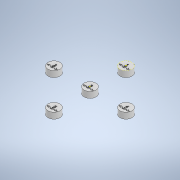
# Autodesk Inventor part: 5-circles-test-print
Saved by Autodesk Inventor 2020.3 (Build 243373000, 373)
## iProperties
Created: 2020-06-02
Part Number: 5-circles-test-print
Material: Generic
Document SubType Name: Modeling
Designer: robst
Density: 1 g/cm^3
Appearance: Default
Author: robst
Autodesk Inventor part; units mm, degrees
ref_plane "YZ Plane" through (0, 0, 0) normal (1, 0, 0) x (0, 1, 0)
ref_plane "XZ Plane" through (0, 0, 0) normal (0, 1, 0) x (-1, 0, 0)
ref_plane "XY Plane" through (0, 0, 0) normal (0, 0, 1) x (1, 0, 0)
sketch "Sketch1" plane through (0, 0, 0) normal (0, 1, 0) x (-1, 0, 0)
  circle A0 centre (0, 0) radius 12.7
  circle A1 centre (76.2, 0) radius 12.7
  circle A2 centre (0, -76.2) radius 12.7
  circle A3 centre (-76.2, 0) radius 12.7
  circle A4 centre (0, 76.2) radius 12.7
  dimension "d0" = 25.4
  dimension "d1" = 76.2
  dimension "d2" = 76.2
  dimension "d3" = 76.2
  dimension "d4" = 76.2
  constraints: 5 centre point, 4 equal radius, 1 coincident
  measures "d0" diameter of A0
  measures "d1" distance of A1.centre point (0, 0)
  measures "d2" distance of A2.centre point (0, 0)
  measures "d3" distance of A3.centre point (0, 0)
  measures "d4" distance of A4.centre point (0, 0)
extrude "Extrusion1" add sketch "Sketch1" along normal blind 12.7
sketch "Sketch4" plane through (0, 12.7, -76.2) normal (0, 1, 0) x (1, 0, 0)
  circle A0 centre (0, 0) radius 12.7 construction
  point P0 (0, -76.2)
sketch "Sketch5" plane through (0, 12.7, 0) normal (0, 1, 0) x (1, 0, 0)
  circle A0 centre (0, 76.2) radius 12.7 construction
  line L0 (-12.7, 76.2) -> (12.7, 76.2) construction
  circle A1 centre (0, 0) radius 12.7 construction
  line L1 (-12.7, 0) -> (12.7, 0) construction
  line L2 (-88.5573, 0) -> (-63.5, 0) construction
  circle A2 centre (-76.2, 0) radius 12.7 construction
  circle A3 centre (76.2, 0) radius 12.7 construction
  line L3 (63.5, 0) -> (88.9, 0) construction
  circle A4 centre (0, -76.2) radius 12.7 construction
  line L4 (-12.7, -76.2) -> (12.7, -76.2) construction
  line L5 (1.7969, 76.2) -> (-1.5582, 76.2)
  line L6 (-1.5582, 76.2) -> (-1.5582, 77.0851)
  line L7 (-1.5582, 77.0851) -> (-0.4878, 77.0851)
  line L8 (-0.4878, 77.0851) -> (-0.4878, 79.7733)
  line L9 (-0.4878, 79.7733) -> (-1.5582, 79.7733)
  line L10 (-1.5582, 79.7733) -> (-1.5582, 80.6007)
  spline S0 degree 2 poles (-1.5582, 80.6007) (-1.3235, 80.6007) (-0.8583, 80.6625) (-0.7184, 80.7284) knots 0 0 0 1 2 2 2
  spline S1 degree 2 poles (-0.7184, 80.7284) (-0.5578, 80.8107) (-0.3767, 81.0865) (-0.3602, 81.2924) knots 0 0 0 1 2 2 2
  line L11 (-0.3602, 81.2924) -> (0.7513, 81.2924)
  line L12 (0.7513, 81.2924) -> (0.7513, 77.0851)
  line L13 (0.7513, 77.0851) -> (1.7969, 77.0851)
  line L14 (1.7969, 77.0851) -> (1.7969, 76.2)
  line L15 (-6.1256, 70.1534) -> (-10.5058, 71.973)
  line L16 (-10.5058, 71.973) -> (-10.5058, 72.7222)
  line L17 (-10.5058, 72.7222) -> (-6.1256, 74.5418)
  line L18 (-6.1256, 74.5418) -> (-6.1256, 73.5991)
  line L19 (-6.1256, 73.5991) -> (-9.1885, 72.3435)
  line L20 (-9.1885, 72.3435) -> (-6.1256, 71.0961)
  line L21 (-6.1256, 71.0961) -> (-6.1256, 70.1534)
  line L22 (-2.7705, 71.8742) -> (-5.0306, 71.8742)
  line L23 (-5.0306, 71.8742) -> (-5.0306, 72.821)
  line L24 (-5.0306, 72.821) -> (-2.7705, 72.821)
  line L25 (-2.7705, 72.821) -> (-2.7705, 71.8742)
  line L26 (2.433, 70.104) -> (0.9592, 70.104)
  line L27 (0.9592, 70.104) -> (-0.0206, 71.7219)
  line L28 (-0.0206, 71.7219) -> (-1.0209, 70.104)
  line L29 (-1.0209, 70.104) -> (-2.433, 70.104)
  line L30 (-2.433, 70.104) -> (-0.7822, 72.6605)
  line L31 (-0.7822, 72.6605) -> (-2.3671, 75.184)
  line L32 (-2.3671, 75.184) -> (-0.8933, 75.184)
  line L33 (-0.8933, 75.184) -> (0.0247, 73.6485)
  line L34 (0.0247, 73.6485) -> (0.9674, 75.184)
  line L35 (0.9674, 75.184) -> (2.3794, 75.184)
  line L36 (2.3794, 75.184) -> (0.7863, 72.714)
  line L37 (0.7863, 72.714) -> (2.433, 70.104)
  line L38 (5.1088, 71.8742) -> (2.8488, 71.8742)
  line L39 (2.8488, 71.8742) -> (2.8488, 72.821)
  line L40 (2.8488, 72.821) -> (5.1088, 72.821)
  line L41 (5.1088, 72.821) -> (5.1088, 71.8742)
  line L42 (10.5881, 71.973) -> (6.208, 70.1534)
  line L43 (6.208, 70.1534) -> (6.208, 71.0961)
  line L44 (6.208, 71.0961) -> (9.2667, 72.3476)
  line L45 (9.2667, 72.3476) -> (6.208, 73.5991)
  line L46 (6.208, 73.5991) -> (6.208, 74.5418)
  line L47 (6.208, 74.5418) -> (10.5881, 72.7222)
  line L48 (10.5881, 72.7222) -> (10.5881, 71.973)
  line L49 (-74.0053, 0) -> (-77.7391, 0)
  line L50 (-77.7391, 0) -> (-77.7391, 0.8275)
  spline S2 degree 2 poles (-77.7391, 0.8275) (-77.2657, 1.2062) (-76.5082, 1.8731) (-76.2242, 2.1736) knots 0 0 0 1 2 2 2
  spline S3 degree 2 poles (-76.2242, 2.1736) (-75.8496, 2.5647) (-75.5161, 3.1616) (-75.5161, 3.4745) knots 0 0 0 1 2 2 2
  spline S4 degree 2 poles (-75.5161, 3.4745) (-75.5161, 3.8285) (-75.9401, 4.2073) (-76.3189, 4.2073) knots 0 0 0 1 2 2 2
  spline S5 degree 2 poles (-76.3189, 4.2073) (-76.5124, 4.2073) (-76.8582, 4.1126) (-77.0352, 4.0385) knots 0 0 0 1 2 2 2
  spline S6 degree 2 poles (-77.0352, 4.0385) (-77.2081, 3.9603) (-77.4551, 3.7956) (-77.5168, 3.7544) knots 0 0 0 1 2 2 2
  line L51 (-77.5168, 3.7544) -> (-77.6156, 3.7544)
  line L52 (-77.6156, 3.7544) -> (-77.6156, 4.8618)
  spline S7 degree 2 poles (-77.6156, 4.8618) (-77.4016, 4.9647) (-76.4877, 5.1788) (-76.0636, 5.1788) knots 0 0 0 1 2 2 2
  spline S8 degree 2 poles (-76.0636, 5.1788) (-75.158, 5.1788) (-74.2276, 4.3719) (-74.2276, 3.6433) knots 0 0 0 1 2 2 2
  spline S9 degree 2 poles (-74.2276, 3.6433) (-74.2276, 3.1946) (-74.6516, 2.33) (-75.1415, 1.836) knots 0 0 0 1 2 2 2
  spline S10 degree 2 poles (-75.1415, 1.836) (-75.4502, 1.5314) (-76.0307, 1.058) (-76.1583, 0.9592) knots 0 0 0 1 2 2 2
  line L53 (-76.1583, 0.9592) -> (-74.0053, 0.9592)
  line L54 (-74.0053, 0.9592) -> (-74.0053, 0)
  line L55 (-82.1543, -6.0466) -> (-86.5344, -4.227)
  line L56 (-86.5344, -4.227) -> (-86.5344, -3.4778)
  line L57 (-86.5344, -3.4778) -> (-82.1543, -1.6582)
  line L58 (-82.1543, -1.6582) -> (-82.1543, -2.6009)
  line L59 (-82.1543, -2.6009) -> (-85.2171, -3.8565)
  line L60 (-85.2171, -3.8565) -> (-82.1543, -5.1039)
  line L61 (-82.1543, -5.1039) -> (-82.1543, -6.0466)
  line L62 (-78.7992, -4.3258) -> (-81.0592, -4.3258)
  line L63 (-81.0592, -4.3258) -> (-81.0592, -3.379)
  line L64 (-81.0592, -3.379) -> (-78.7992, -3.379)
  line L65 (-78.7992, -3.379) -> (-78.7992, -4.3258)
  line L66 (-73.5957, -6.096) -> (-75.0695, -6.096)
  line L67 (-75.0695, -6.096) -> (-76.0492, -4.4781)
  line L68 (-76.0492, -4.4781) -> (-77.0496, -6.096)
  line L69 (-77.0496, -6.096) -> (-78.4616, -6.096)
  line L70 (-78.4616, -6.096) -> (-76.8108, -3.5395)
  line L71 (-76.8108, -3.5395) -> (-78.3957, -1.016)
  line L72 (-78.3957, -1.016) -> (-76.922, -1.016)
  line L73 (-76.922, -1.016) -> (-76.0039, -2.5515)
  line L74 (-76.0039, -2.5515) -> (-75.0612, -1.016)
  line L75 (-75.0612, -1.016) -> (-73.6492, -1.016)
  line L76 (-73.6492, -1.016) -> (-75.2424, -3.486)
  line L77 (-75.2424, -3.486) -> (-73.5957, -6.096)
  line L78 (-70.9198, -4.3258) -> (-73.1799, -4.3258)
  line L79 (-73.1799, -4.3258) -> (-73.1799, -3.379)
  line L80 (-73.1799, -3.379) -> (-70.9198, -3.379)
  line L81 (-70.9198, -3.379) -> (-70.9198, -4.3258)
  line L82 (-65.4405, -4.227) -> (-69.8207, -6.0466)
  line L83 (-69.8207, -6.0466) -> (-69.8207, -5.1039)
  line L84 (-69.8207, -5.1039) -> (-66.762, -3.8524)
  line L85 (-66.762, -3.8524) -> (-69.8207, -2.6009)
  line L86 (-69.8207, -2.6009) -> (-69.8207, -1.6582)
  line L87 (-69.8207, -1.6582) -> (-65.4405, -3.4778)
  line L88 (-65.4405, -3.4778) -> (-65.4405, -4.227)
  spline S11 degree 2 poles (1.8957, 1.5396) (1.8957, 1.165) (1.6199, 0.5516) (1.3523, 0.3376) knots 0 0 0 1 2 2 2
  spline S12 degree 2 poles (1.3523, 0.3376) (1.0847, 0.1235) (0.3561, -0.107) (-0.1667, -0.107) knots 0 0 0 1 2 2 2
  spline S13 degree 2 poles (-0.1667, -0.107) (-0.7595, -0.107) (-1.6076, 0.0906) (-1.8752, 0.2141) knots 0 0 0 1 2 2 2
  line L89 (-1.8752, 0.2141) -> (-1.8752, 1.3173)
  line L90 (-1.8752, 1.3173) -> (-1.7517, 1.3173)
  spline S14 degree 2 poles (-1.7517, 1.3173) (-1.4717, 1.1403) (-0.7184, 0.8769) (-0.4055, 0.8769) knots 0 0 0 1 2 2 2
  spline S15 degree 2 poles (-0.4055, 0.8769) (-0.2202, 0.8769) (0.212, 0.9427) (0.3602, 1.0498) knots 0 0 0 1 2 2 2
  spline S16 degree 2 poles (0.3602, 1.0498) (0.4755, 1.1362) (0.6154, 1.3873) (0.6154, 1.6137) knots 0 0 0 1 2 2 2
  spline S17 degree 2 poles (0.6154, 1.6137) (0.6154, 1.8402) (0.4178, 2.083) (0.2532, 2.1407) knots 0 0 0 1 2 2 2
  spline S18 degree 2 poles (0.2532, 2.1407) (0.0885, 2.1983) (-0.3684, 2.2107) (-0.5455, 2.2107) knots 0 0 0 1 2 2 2
  line L91 (-0.5455, 2.2107) -> (-0.7636, 2.2107)
  line L92 (-0.7636, 2.2107) -> (-0.7636, 3.104)
  line L93 (-0.7636, 3.104) -> (-0.5619, 3.104)
  spline S19 degree 2 poles (-0.5619, 3.104) (-0.3314, 3.104) (0.0597, 3.1452) (0.1955, 3.2069) knots 0 0 0 1 2 2 2
  spline S20 degree 2 poles (0.1955, 3.2069) (0.3314, 3.2728) (0.4837, 3.5033) (0.4837, 3.7009) knots 0 0 0 1 2 2 2
  spline S21 degree 2 poles (0.4837, 3.7009) (0.4837, 3.8573) (0.3396, 4.0508) (0.2367, 4.1043) knots 0 0 0 1 2 2 2
  spline S22 degree 2 poles (0.2367, 4.1043) (0.1132, 4.1661) (-0.2161, 4.2073) (-0.3314, 4.2073) knots 0 0 0 1 2 2 2
  spline S23 degree 2 poles (-0.3314, 4.2073) (-0.5166, 4.2073) (-0.9077, 4.1208) (-1.0889, 4.0508) knots 0 0 0 1 2 2 2
  spline S24 degree 2 poles (-1.0889, 4.0508) (-1.2329, 3.9973) (-1.5458, 3.8244) (-1.6199, 3.7791) knots 0 0 0 1 2 2 2
  line L94 (-1.6199, 3.7791) -> (-1.727, 3.7791)
  line L95 (-1.727, 3.7791) -> (-1.727, 4.8659)
  spline S25 degree 2 poles (-1.727, 4.8659) (-1.4635, 4.9771) (-0.5743, 5.187) (-0.1091, 5.187) knots 0 0 0 1 2 2 2
  spline S26 degree 2 poles (-0.1091, 5.187) (0.3437, 5.187) (1.0106, 5.0306) (1.2453, 4.8783) knots 0 0 0 1 2 2 2
  spline S27 degree 2 poles (1.2453, 4.8783) (1.5047, 4.7177) (1.764, 4.2237) (1.764, 3.915) knots 0 0 0 1 2 2 2
  spline S28 degree 2 poles (1.764, 3.915) (1.764, 3.4786) (1.2618, 2.8282) (0.8501, 2.7335) knots 0 0 0 1 2 2 2
  line L96 (0.8501, 2.7335) -> (0.8501, 2.6841)
  spline S29 degree 2 poles (0.8501, 2.6841) (1.0312, 2.6594) (1.377, 2.5276) (1.5417, 2.3794) knots 0 0 0 1 2 2 2
  spline S30 degree 2 poles (1.5417, 2.3794) (1.694, 2.2477) (1.8957, 1.8278) (1.8957, 1.5396) knots 0 0 0 1 2 2 2
  line L97 (-6.1256, -6.0466) -> (-10.5058, -4.227)
  line L98 (-10.5058, -4.227) -> (-10.5058, -3.4778)
  line L99 (-10.5058, -3.4778) -> (-6.1256, -1.6582)
  line L100 (-6.1256, -1.6582) -> (-6.1256, -2.6009)
  line L101 (-6.1256, -2.6009) -> (-9.1885, -3.8565)
  line L102 (-9.1885, -3.8565) -> (-6.1256, -5.1039)
  line L103 (-6.1256, -5.1039) -> (-6.1256, -6.0466)
  line L104 (-2.7705, -4.3258) -> (-5.0306, -4.3258)
  line L105 (-5.0306, -4.3258) -> (-5.0306, -3.379)
  line L106 (-5.0306, -3.379) -> (-2.7705, -3.379)
  line L107 (-2.7705, -3.379) -> (-2.7705, -4.3258)
  line L108 (2.433, -6.096) -> (0.9592, -6.096)
  line L109 (0.9592, -6.096) -> (-0.0206, -4.4781)
  line L110 (-0.0206, -4.4781) -> (-1.0209, -6.096)
  line L111 (-1.0209, -6.096) -> (-2.433, -6.096)
  line L112 (-2.433, -6.096) -> (-0.7822, -3.5395)
  line L113 (-0.7822, -3.5395) -> (-2.3671, -1.016)
  line L114 (-2.3671, -1.016) -> (-0.8933, -1.016)
  line L115 (-0.8933, -1.016) -> (0.0247, -2.5515)
  line L116 (0.0247, -2.5515) -> (0.9674, -1.016)
  line L117 (0.9674, -1.016) -> (2.3794, -1.016)
  line L118 (2.3794, -1.016) -> (0.7863, -3.486)
  line L119 (0.7863, -3.486) -> (2.433, -6.096)
  line L120 (5.1088, -4.3258) -> (2.8488, -4.3258)
  line L121 (2.8488, -4.3258) -> (2.8488, -3.379)
  line L122 (2.8488, -3.379) -> (5.1088, -3.379)
  line L123 (5.1088, -3.379) -> (5.1088, -4.3258)
  line L124 (10.5881, -4.227) -> (6.208, -6.0466)
  line L125 (6.208, -6.0466) -> (6.208, -5.1039)
  line L126 (6.208, -5.1039) -> (9.2667, -3.8524)
  line L127 (9.2667, -3.8524) -> (6.208, -2.6009)
  line L128 (6.208, -2.6009) -> (6.208, -1.6582)
  line L129 (6.208, -1.6582) -> (10.5881, -3.4778)
  line L130 (10.5881, -3.4778) -> (10.5881, -4.227)
  line L131 (78.2851, 1.1856) -> (77.5976, 1.1856)
  line L132 (77.5976, 1.1856) -> (77.5976, -0.0124)
  line L133 (77.5976, -0.0124) -> (76.3667, -0.0124)
  line L134 (76.3667, -0.0124) -> (76.3667, 1.1856)
  line L135 (76.3667, 1.1856) -> (74.1272, 1.1856)
  line L136 (74.1272, 1.1856) -> (74.1272, 2.1324)
  line L137 (74.1272, 2.1324) -> (76.3256, 5.08)
  line L138 (76.3256, 5.08) -> (77.5976, 5.08)
  line L139 (77.5976, 5.08) -> (77.5976, 2.0995)
  line L140 (77.5976, 2.0995) -> (78.2851, 2.0995)
  line L141 (78.2851, 2.0995) -> (78.2851, 1.1856)
  line L142 (76.3667, 2.0995) -> (76.3667, 3.8285)
  line L143 (76.3667, 3.8285) -> (75.0782, 2.0995)
  line L144 (75.0782, 2.0995) -> (76.3667, 2.0995)
  line L145 (70.0744, -6.0466) -> (65.6942, -4.227)
  line L146 (65.6942, -4.227) -> (65.6942, -3.4778)
  line L147 (65.6942, -3.4778) -> (70.0744, -1.6582)
  line L148 (70.0744, -1.6582) -> (70.0744, -2.6009)
  line L149 (70.0744, -2.6009) -> (67.0115, -3.8565)
  line L150 (67.0115, -3.8565) -> (70.0744, -5.1039)
  line L151 (70.0744, -5.1039) -> (70.0744, -6.0466)
  line L152 (73.4295, -4.3258) -> (71.1694, -4.3258)
  line L153 (71.1694, -4.3258) -> (71.1694, -3.379)
  line L154 (71.1694, -3.379) -> (73.4295, -3.379)
  line L155 (73.4295, -3.379) -> (73.4295, -4.3258)
  line L156 (78.633, -6.096) -> (77.1592, -6.096)
  line L157 (77.1592, -6.096) -> (76.1794, -4.4781)
  line L158 (76.1794, -4.4781) -> (75.1791, -6.096)
  line L159 (75.1791, -6.096) -> (73.767, -6.096)
  line L160 (73.767, -6.096) -> (75.4178, -3.5395)
  line L161 (75.4178, -3.5395) -> (73.8329, -1.016)
  line L162 (73.8329, -1.016) -> (75.3067, -1.016)
  line L163 (75.3067, -1.016) -> (76.2247, -2.5515)
  line L164 (76.2247, -2.5515) -> (77.1674, -1.016)
  line L165 (77.1674, -1.016) -> (78.5794, -1.016)
  line L166 (78.5794, -1.016) -> (76.9863, -3.486)
  line L167 (76.9863, -3.486) -> (78.633, -6.096)
  line L168 (81.3088, -4.3258) -> (79.0488, -4.3258)
  line L169 (79.0488, -4.3258) -> (79.0488, -3.379)
  line L170 (79.0488, -3.379) -> (81.3088, -3.379)
  line L171 (81.3088, -3.379) -> (81.3088, -4.3258)
  line L172 (86.7881, -4.227) -> (82.408, -6.0466)
  line L173 (82.408, -6.0466) -> (82.408, -5.1039)
  line L174 (82.408, -5.1039) -> (85.4667, -3.8524)
  line L175 (85.4667, -3.8524) -> (82.408, -2.6009)
  line L176 (82.408, -2.6009) -> (82.408, -1.6582)
  line L177 (82.408, -1.6582) -> (86.7881, -3.4778)
  line L178 (86.7881, -3.4778) -> (86.7881, -4.227)
  spline S31 degree 2 poles (1.9081, -74.4792) (1.9081, -74.8785) (1.6364, -75.5537) (1.3688, -75.7966) knots 0 0 0 1 2 2 2
  spline S32 degree 2 poles (1.3688, -75.7966) (1.1012, -76.0394) (0.3684, -76.307) (-0.1667, -76.307) knots 0 0 0 1 2 2 2
  spline S33 degree 2 poles (-0.1667, -76.307) (-0.7348, -76.3029) (-1.5499, -76.1177) (-1.8175, -75.9983) knots 0 0 0 1 2 2 2
  line L179 (-1.8175, -75.9983) -> (-1.8175, -74.8909)
  line L180 (-1.8175, -74.8909) -> (-1.7023, -74.8909)
  spline S34 degree 2 poles (-1.7023, -74.8909) (-1.6035, -74.9444) (-1.3647, -75.0844) (-1.1712, -75.1585) knots 0 0 0 1 2 2 2
  spline S35 degree 2 poles (-1.1712, -75.1585) (-0.9901, -75.2285) (-0.6154, -75.3231) (-0.389, -75.3231) knots 0 0 0 1 2 2 2
  spline S36 degree 2 poles (-0.389, -75.3231) (-0.1914, -75.3231) (0.2696, -75.2243) (0.4096, -75.0926) knots 0 0 0 1 2 2 2
  spline S37 degree 2 poles (0.4096, -75.0926) (0.5125, -74.9897) (0.6278, -74.7386) (0.6278, -74.5286) knots 0 0 0 1 2 2 2
  spline S38 degree 2 poles (0.6278, -74.5286) (0.6278, -74.3475) (0.4796, -74.0923) (0.3602, -74.014) knots 0 0 0 1 2 2 2
  spline S39 degree 2 poles (0.3602, -74.014) (0.1873, -73.8988) (-0.3067, -73.8329) (-0.4837, -73.8329) knots 0 0 0 1 2 2 2
  spline S40 degree 2 poles (-0.4837, -73.8329) (-0.7636, -73.8329) (-1.2947, -73.9235) (-1.4882, -73.9729) knots 0 0 0 1 2 2 2
  line L181 (-1.4882, -73.9729) -> (-1.5993, -73.9729)
  line L182 (-1.5993, -73.9729) -> (-1.5993, -71.12)
  line L183 (-1.5993, -71.12) -> (1.7681, -71.12)
  line L184 (1.7681, -71.12) -> (1.7681, -72.0792)
  line L185 (1.7681, -72.0792) -> (-0.3931, -72.0792)
  line L186 (-0.3931, -72.0792) -> (-0.3931, -72.9231)
  spline S41 degree 2 poles (-0.3931, -72.9231) (-0.2902, -72.9149) (-0.0062, -72.9066) (0.072, -72.9066) knots 0 0 0 1 2 2 2
  spline S42 degree 2 poles (0.072, -72.9066) (0.4384, -72.9066) (1.0559, -73.0548) (1.2988, -73.2072) knots 0 0 0 1 2 2 2
  spline S43 degree 2 poles (1.2988, -73.2072) (1.587, -73.3965) (1.9081, -74.0264) (1.9081, -74.4792) knots 0 0 0 1 2 2 2
  line L187 (-6.1256, -82.2466) -> (-10.5058, -80.427)
  line L188 (-10.5058, -80.427) -> (-10.5058, -79.6778)
  line L189 (-10.5058, -79.6778) -> (-6.1256, -77.8582)
  line L190 (-6.1256, -77.8582) -> (-6.1256, -78.8009)
  line L191 (-6.1256, -78.8009) -> (-9.1885, -80.0565)
  line L192 (-9.1885, -80.0565) -> (-6.1256, -81.3039)
  line L193 (-6.1256, -81.3039) -> (-6.1256, -82.2466)
  line L194 (-2.7705, -80.5258) -> (-5.0306, -80.5258)
  line L195 (-5.0306, -80.5258) -> (-5.0306, -79.579)
  line L196 (-5.0306, -79.579) -> (-2.7705, -79.579)
  line L197 (-2.7705, -79.579) -> (-2.7705, -80.5258)
  line L198 (2.433, -82.296) -> (0.9592, -82.296)
  line L199 (0.9592, -82.296) -> (-0.0206, -80.6781)
  line L200 (-0.0206, -80.6781) -> (-1.0209, -82.296)
  line L201 (-1.0209, -82.296) -> (-2.433, -82.296)
  line L202 (-2.433, -82.296) -> (-0.7822, -79.7395)
  line L203 (-0.7822, -79.7395) -> (-2.3671, -77.216)
  line L204 (-2.3671, -77.216) -> (-0.8933, -77.216)
  line L205 (-0.8933, -77.216) -> (0.0247, -78.7515)
  line L206 (0.0247, -78.7515) -> (0.9674, -77.216)
  line L207 (0.9674, -77.216) -> (2.3794, -77.216)
  line L208 (2.3794, -77.216) -> (0.7863, -79.686)
  line L209 (0.7863, -79.686) -> (2.433, -82.296)
  line L210 (5.1088, -80.5258) -> (2.8488, -80.5258)
  line L211 (2.8488, -80.5258) -> (2.8488, -79.579)
  line L212 (2.8488, -79.579) -> (5.1088, -79.579)
  line L213 (5.1088, -79.579) -> (5.1088, -80.5258)
  line L214 (10.5881, -80.427) -> (6.208, -82.2466)
  line L215 (6.208, -82.2466) -> (6.208, -81.3039)
  line L216 (6.208, -81.3039) -> (9.2667, -80.0524)
  line L217 (9.2667, -80.0524) -> (6.208, -78.8009)
  line L218 (6.208, -78.8009) -> (6.208, -77.8582)
  line L219 (6.208, -77.8582) -> (10.5881, -79.6778)
  line L220 (10.5881, -79.6778) -> (10.5881, -80.427)
  constraints: 12 horizontal, 10 end point, 8 point on circle, 2 point on line, 1 horizontal alignment, 1 parallel, 1 other
extrude "Extrusion4" cut sketch "Sketch5" against normal blind 5.08
body "Solid1"
